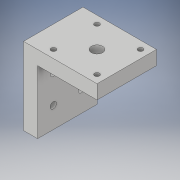
# Autodesk Inventor part: Stepper_Face
Saved by Autodesk Inventor 2019 (Build 230136000, 136)
## iProperties
Created: 2019-07-06
Part Number: Stepper_Face
Material: Generic
Document SubType Name: Modeling
Designer: Jorian Brusind
Density: 1 g/cm^3
Appearance: Default
Author: Jorian Brusind
Autodesk Inventor part; units mm, degrees
ref_plane "YZ Plane" through (0, 0, 0) normal (1, 0, 0) x (0, 1, 0)
ref_plane "XZ Plane" through (0, 0, 0) normal (0, 1, 0) x (-1, 0, 0)
ref_plane "XY Plane" through (0, 0, 0) normal (0, 0, 1) x (1, 0, 0)
sketch "Sketch1" plane through (0, 0, 0) normal (0, 1, 0) x (-1, 0, 0)
  line L0 (0, 0) -> (52.3, 0)
  line L1 (52.3, 0) -> (52.3, -42.3)
  line L2 (52.3, -42.3) -> (0, -42.3)
  line L3 (0, -42.3) -> (0, 0)
  dimension "d0" = 52.3
  dimension "d1" = 42.3
  constraints: 8 end point, 2 parallel, 1 horizontal, 1 perpendicular
  measures "d0" distance of L1.end L2.end
  measures "d1" distance of L0.end L1.end
extrude "Extrusion1" add sketch "Sketch1" along normal blind 10
sketch "Sketch2" plane through (0, 0, 0) normal (0, -1, 0) x (1, 0, 0)
  line L0 (-52.3, 0) -> (0, 0) projected
  line L1 (-52.3, 0) -> (-42.3, 0)
  line L2 (-42.3, 0) -> (-42.3, -42.3)
  line L3 (-42.3, -42.3) -> (-52.3, -42.3)
  line L4 (-52.3, -42.3) -> (-52.3, 0)
  dimension "d4" = 10
  dimension "d5" = 42.3
  constraints: 8 end point, 2 parallel, 1 horizontal, 1 perpendicular
  measures "d4" distance of L2.end L3.end
  measures "d5" distance of L1.end L2.end
extrude "Extrusion2" add sketch "Sketch2" along normal blind 45
sketch "Sketch3" plane through (0, 10, 0) normal (0, 1, 0) x (1, 0, 0)
  line L0 (0, 0) -> (0, 5.65)
  line L1 (0, 0) -> (0, 42.3) projected
  line L2 (0, 5.65) -> (-5.65, 5.65)
  circle A0 centre (-5.65, 5.65) radius 1.75
  circle A1 centre (-5.65, 36.65) radius 1.75
  circle A2 centre (-36.65, 5.65) radius 1.75
  circle A3 centre (-36.65, 36.65) radius 1.75
  dimension "d8" = 5.65
  dimension "d9" = 5.65
  dimension "d10" = 3.5
  dimension "d13" = 31
  dimension "d16" = 31
  constraints: 4 centre point, 4 end point, 1 coincident, 1 horizontal, 1 perpendicular, 1 point on line, 1 vertical, 6 other
  measures "d8" distance of L0.start L0.end
  measures "d9" distance of L0.end L2.end
  measures "d10" diameter of A0
  measures "d13" distance of A0.centre A1.centre
  measures "d16" distance of A0.centre A2.centre
extrude "Extrusion3" cut sketch "Sketch3" against normal blind 10
sketch "Sketch4" plane through (0, 10, 0) normal (0, 1, 0) x (1, 0, 0)
  line L0 (0, 42.3) -> (0, 0) projected
  line L1 (0, 21.15) -> (-21.15, 21.15)
  circle A0 centre (-21.15, 21.15) radius 4
  dimension "d21" = 21.15
  dimension "d22" = 8
  constraints: 2 end point, 1 centre point, 1 coincident, 1 horizontal, 1 midpoint
  measures "d21" distance of L1.start L1.end
  measures "d22" diameter of A0
extrude "Extrusion4" cut sketch "Sketch4" against normal blind 10
sketch "Sketch5" plane through (-52.3, 10, -42.3) normal (-1, 0, 0) x (0, 0, 1)
  line L0 (0, -55) -> (42.3, -55) projected
  line L1 (25.15, -10) -> (17.15, -10) projected
  line L2 (21.15, -55) -> (11.15, -55)
  line L3 (11.15, -55) -> (11.15, -40)
  circle A0 centre (11.15, -40) radius 2.25
  circle A1 centre (31.15, -40) radius 2.25
  circle A2 centre (11.15, -20) radius 2.25
  circle A3 centre (31.15, -20) radius 2.25
  point P0 (42.3, -10)
  dimension "d30" = 10
  dimension "d31" = 15
  dimension "d32" = 4.5
  dimension "d35" = 20
  dimension "d38" = 20
  constraints: 4 centre point, 4 end point, 1 coincident, 1 horizontal, 1 midpoint, 1 perpendicular, 1 point on line, 1 vertical, 6 other
  measures "d30" distance of L2.start L2.end
  measures "d31" distance of L2.end L3.end
  measures "d32" diameter of A0
  measures "d35" distance of A0.centre A1.centre
  measures "d38" distance of A0.centre A2.centre
extrude "Extrusion5" cut sketch "Sketch5" against normal blind 10
body "Solid1"
